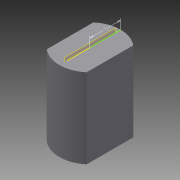
# Autodesk Inventor part: Pieza3
Saved by Autodesk Inventor 2013 (Build 170138000, 138)
## iProperties
Created: 2014-07-04
Part Number: Pieza3
Material: Genérico
Document SubType Name: Chapa
Designer: Administrador
Density: 1 g/cm^3
Sheet Metal Rule: Por defecto_mm
Author: Administrador
Autodesk Inventor part; units mm, degrees
ref_plane "YZ Plane" through (0, 0, 0) normal (1, 0, 0) x (0, 1, 0)
ref_plane "XZ Plane" through (0, 0, 0) normal (0, 1, 0) x (-1, 0, 0)
ref_plane "XY Plane" through (0, 0, 0) normal (0, 0, 1) x (1, 0, 0)
sketch "Boceto3" plane through (0, 0, 0) normal (0, 0, 1) x (1, 0, 0)
  line L0 (-13, 21.9872) -> (13, 21.9872)
  line L1 (13, 21.9872) -> (13, -21.9872)
  line L2 (13, -21.9872) -> (-13, -21.9872)
  line L3 (-13, -21.9872) -> (-13, 21.9872)
  line L4 (-13, 21.9872) -> (13, -21.9872) construction
  line L5 (13, 21.9872) -> (-13, -21.9872) construction
  line L6 (-11, 21.2441) -> (11, 21.2441)
  line L7 (11, -21.2441) -> (-11, -21.2441)
  line L8 (-11, 21.2441) -> (11, -21.2441) construction
  line L9 (11, 21.2441) -> (-11, -21.2441) construction
  line L10 (-11, 16.7033) -> (-11, 21.2441)
  line L11 (11, 21.2441) -> (11, 16.7033)
  arc A0 (11, 14.2478) -> (-11, 14.2478) centre (0, 0) ccw
  line L12 (11, 14.2478) -> (11, -14.2478)
  line L13 (11, -16.7033) -> (11, -21.2441)
  line L14 (-11, -21.2441) -> (-11, -16.7033)
  line L15 (-11, -14.2478) -> (-11, 14.2478)
  arc A1 (-11, -14.2478) -> (11, -14.2478) centre (0, 0) ccw
  arc A2 (13, 15.1987) -> (-13, 15.1987) centre (0, 0) ccw
  arc A3 (-13, -15.1987) -> (13, -15.1987) centre (0, 0) ccw
  dimension "d11" = 26
  dimension "d12" = 22
  constraints: 32 end point, 12 parallel, 12 point on circle, 4 centre point, 4 midpoint, 4 perpendicular, 4 point on line, 2 horizontal
  measures "d11" distance of L1.end L2.end
  measures "d12" distance of L7.start L7.end
extrude "Extrusión2" add sketch "Boceto3" along normal blind 50 contours A2 L1 A3 L3
sketch "Boceto5" plane through (0, 0, 50) normal (0, 0, 1) x (1, 0, 0)
  arc A0 (13, 15.1987) -> (-13, 15.1987) centre (0, 0) ccw projected
  line L0 (-13, 15.1987) -> (-13, -15.1987) projected
  arc A1 (-13, -15.1987) -> (13, -15.1987) centre (0, 0) ccw projected
  line L1 (13, -15.1987) -> (13, 15.1987) projected
extrude "Extrusión3" add sketch "Boceto5" along normal blind 2
ref_plane "Plano de trabajo1" through (0, -15.1987, 0) normal (1, 0, 0) x (0, 0, -1)
sketch "Boceto6" plane through (0, -15.1987, 0) normal (1, 0, 0) x (0, 0, -1)
  line L0 (-52, 0) -> (-52, 30.3974) projected
  line L1 (-52, 15.1987) -> (-52, 35.1987)
  point P0 (0, 15.1987)
  dimension "d18" = 20
  constraints: 2 end point
  measures "d18" distance of L1.start L1.end
equation "\"Radio_pliegue\" = Grosor"
equation "\"Anchura_desahogo_plegado\" = Grosor"
equation "\"Profundidad_desahogo_plegado\" = 0.5 * Grosor"
equation "\"Tamaño_destalonado\" = 4 * Grosor"
equation "\"Remanente_mínimo\" = 2 * Grosor"
equation "\"Radiodetransición\" = Radio_pliegue"
equation "\"Tamaño_de_radio_de_Jacobi\" = Radio_pliegue"
equation "\"TamañoSeparación\" = Grosor"
equation "\"Grosor\" = 0.5"
